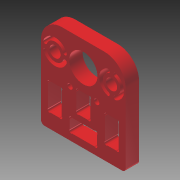
# Autodesk Inventor part: gantry2
Saved by Autodesk Inventor 2012 SP1 (Build 160190100, 190)
## iProperties
Created: 2011-10-14
Part Number: gantry2
Document SubType Name: Modeling
Designer: cramera
Density: 0.952 g/cm^3
Material: High Density Polyethylene
Mass: 45.0071 g
Surface Area: 204.192 cm^2
Volume: 47.2763 cm^3
Autodesk Inventor part; units mm, degrees
ref_plane "YZ Plane" through (0, 0, 0) normal (1, 0, 0) x (0, 1, 0)
ref_plane "XZ Plane" through (0, 0, 0) normal (0, 1, 0) x (-1, 0, 0)
ref_plane "XY Plane" through (0, 0, 0) normal (0, 0, 1) x (1, 0, 0)
derived "skeleton.ipt"
sketch "DRILL-THROUGH" plane through (0, 0, 0) normal (0, 0, 1) x (1, 0, 0)
  arc A0 (596.6867, 478.8812) -> (598.2742, 477.2937) centre (598.2742, 478.8812) ccw
  arc A1 (598.2742, 508.2817) -> (599.8617, 509.8692) centre (598.2742, 509.8692) ccw
  arc A2 (599.8617, 509.8692) -> (598.2742, 511.4567) centre (598.2742, 509.8692) ccw
  arc A3 (598.2742, 511.4567) -> (596.6867, 509.8692) centre (598.2742, 509.8692) ccw
  arc A4 (596.6867, 509.8692) -> (598.2742, 508.2817) centre (598.2742, 509.8692) ccw
  arc A5 (629.2622, 508.2817) -> (630.8497, 509.8692) centre (629.2622, 509.8692) ccw
  arc A6 (630.8497, 509.8692) -> (629.2622, 511.4567) centre (629.2622, 509.8692) ccw
  arc A7 (629.2622, 511.4567) -> (627.6747, 509.8692) centre (629.2622, 509.8692) ccw
  arc A8 (627.6747, 509.8692) -> (629.2622, 508.2817) centre (629.2622, 509.8692) ccw
  arc A9 (599.8617, 478.8812) -> (598.2742, 480.4687) centre (598.2742, 478.8812) ccw
  arc A10 (598.2742, 477.2937) -> (599.8617, 478.8812) centre (598.2742, 478.8812) ccw
  arc A11 (598.2742, 480.4687) -> (596.6867, 478.8812) centre (598.2742, 478.8812) ccw
  arc A12 (630.8497, 478.8812) -> (629.2622, 480.4687) centre (629.2622, 478.8812) ccw
  arc A13 (629.2622, 477.2937) -> (630.8497, 478.8812) centre (629.2622, 478.8812) ccw
  arc A14 (627.6747, 478.8812) -> (629.2622, 477.2937) centre (629.2622, 478.8812) ccw
  arc A15 (629.2622, 480.4687) -> (627.6747, 478.8812) centre (629.2622, 478.8812) ccw
  constraints: 32 point on circle, 16 centre point
sketch "POCKET_3-8" plane through (0, 0, 0) normal (0, 0, 1) x (1, 0, 0)
  circle A0 centre (625.7697, 474.1185) radius 6.0458
  circle A1 centre (601.7667, 474.1185) radius 6.0458
  constraints: 2 centre point
sketch "STOCK_12MM" plane through (0, 0, 0) normal (0, 0, 1) x (1, 0, 0)
  line L0 (457.2, 0) -> (914.4, 0)
  line L1 (914.4, 0) -> (914.4, 914.4)
  line L2 (914.4, 914.4) -> (457.2, 914.4)
  line L3 (457.2, 914.4) -> (457.2, 0)
  line L4 (0, 0) -> (457.2, 0)
  line L5 (457.2, 0) -> (457.2, 914.4)
  line L6 (457.2, 914.4) -> (0, 914.4)
  line L7 (0, 914.4) -> (0, 0)
  constraints: 16 end point
sketch "THROUGH-CUT" plane through (0, 0, 0) normal (0, 0, 1) x (1, 0, 0)
  arc A0 (643.0324, 504.8484) -> (640.8954, 503.359) centre (642.4829, 503.359) ccw
  line L0 (640.8954, 503.359) -> (640.8954, 503.2506)
  arc A1 (640.8954, 503.2506) -> (641.9274, 501.7635) centre (642.4829, 503.2506) ccw
  arc A2 (641.9274, 486.9869) -> (641.9274, 501.7635) centre (639.1682, 494.3752) ccw
  arc A3 (641.9274, 486.9869) -> (640.8954, 485.4998) centre (642.4829, 485.4998) ccw
  line L1 (640.8954, 485.4998) -> (640.8954, 485.3914)
  arc A4 (575.6682, 435.1284) -> (578.8432, 431.9534) centre (578.8432, 435.1284) ccw
  line L2 (578.8432, 431.9534) -> (648.6932, 431.9534)
  arc A5 (648.6932, 431.9534) -> (651.8682, 435.1284) centre (648.6932, 435.1284) ccw
  line L3 (651.8682, 435.1284) -> (651.8682, 497.5502)
  arc A6 (651.8682, 497.5502) -> (632.8182, 516.6002) centre (632.8182, 497.5502) ccw
  line L4 (632.8182, 516.6002) -> (594.7182, 516.6002)
  arc A7 (594.7182, 516.6002) -> (575.6682, 497.5502) centre (594.7182, 497.5502) ccw
  line L5 (575.6682, 497.5502) -> (575.6682, 435.1284)
  line L6 (607.6087, 473.0801) -> (607.6087, 458.2663)
  arc A8 (607.6087, 458.2663) -> (609.8537, 456.0212) centre (608.7312, 457.1437) ccw
  line L7 (609.8537, 456.0212) -> (617.6826, 456.0212)
  arc A9 (617.6826, 456.0212) -> (619.9277, 458.2663) centre (618.8051, 457.1437) ccw
  line L8 (619.9277, 458.2663) -> (619.9277, 473.0801)
  arc A10 (619.9277, 473.0801) -> (617.6826, 475.3252) centre (618.8051, 474.2027) ccw
  line L9 (617.6826, 475.3252) -> (609.8537, 475.3252)
  arc A11 (609.8537, 475.3252) -> (607.6087, 473.0801) centre (608.7312, 474.2027) ccw
  arc A12 (601.5762, 440.5485) -> (603.8212, 438.3034) centre (602.6987, 439.426) ccw
  line L10 (603.8212, 438.3034) -> (623.7151, 438.3034)
  arc A13 (623.7151, 438.3034) -> (625.9602, 440.5485) centre (624.8376, 439.426) ccw
  line L11 (625.9602, 440.5485) -> (625.9602, 448.3774)
  arc A14 (625.9602, 448.3774) -> (623.7151, 450.6224) centre (624.8376, 449.4999) ccw
  line L12 (623.7151, 450.6224) -> (603.8212, 450.6224)
  arc A15 (603.8212, 450.6224) -> (601.5762, 448.3774) centre (602.6987, 449.4999) ccw
  line L13 (601.5762, 448.3774) -> (601.5762, 440.5485)
  arc A16 (582.0182, 447.122) -> (582.0182, 444.877) centre (583.1407, 445.9995) ccw
  arc A17 (597.2436, 492.648) -> (595.7564, 491.6159) centre (597.2436, 491.0605) ccw
  line L14 (584.2632, 444.877) -> (592.0921, 444.877)
  arc A18 (592.0921, 444.877) -> (594.3372, 447.122) centre (593.2146, 445.9995) ccw
  line L15 (594.3372, 447.122) -> (594.3372, 467.0159)
  arc A19 (594.3372, 467.0159) -> (592.0921, 469.261) centre (593.2146, 468.1384) ccw
  line L16 (592.0921, 469.261) -> (584.2632, 469.261)
  arc A20 (584.2632, 469.261) -> (582.0182, 469.261) centre (583.1407, 468.1384) ccw
  arc A21 (582.0182, 469.261) -> (582.0182, 467.0159) centre (583.1407, 468.1384) ccw
  line L17 (582.0182, 467.0159) -> (582.0182, 447.122)
  arc A22 (633.1992, 447.122) -> (635.4442, 444.877) centre (634.3217, 445.9995) ccw
  line L18 (635.4442, 444.877) -> (643.2731, 444.877)
  arc A23 (643.2731, 444.877) -> (645.5182, 447.122) centre (644.3956, 445.9995) ccw
  line L19 (645.5182, 447.122) -> (645.5182, 467.0159)
  arc A24 (645.5182, 467.0159) -> (643.2731, 469.261) centre (644.3956, 468.1384) ccw
  line L20 (643.2731, 469.261) -> (635.4442, 469.261)
  arc A25 (635.4442, 469.261) -> (633.1992, 467.0159) centre (634.3217, 468.1384) ccw
  line L21 (633.1992, 467.0159) -> (633.1992, 447.122)
  arc A26 (601.0682, 494.3752) -> (613.7682, 481.6752) centre (613.7682, 494.3752) ccw
  arc A27 (613.7682, 481.6752) -> (626.4682, 494.3752) centre (613.7682, 494.3752) ccw
  arc A28 (626.4682, 494.3752) -> (613.7682, 507.0752) centre (613.7682, 494.3752) ccw
  arc A29 (613.7682, 507.0752) -> (601.0682, 494.3752) centre (613.7682, 494.3752) ccw
  arc A30 (601.7667, 476.5315) -> (599.3537, 474.1185) centre (601.7667, 474.1185) ccw
  arc A31 (599.3537, 474.1185) -> (601.7667, 471.7055) centre (601.7667, 474.1185) ccw
  arc A32 (601.7667, 471.7055) -> (604.1797, 474.1185) centre (601.7667, 474.1185) ccw
  arc A33 (604.1797, 474.1185) -> (601.7667, 476.5315) centre (601.7667, 474.1185) ccw
  arc A34 (597.352, 496.1024) -> (598.8413, 498.2394) centre (597.352, 497.6899) ccw
  arc A35 (598.8413, 498.2394) -> (577.895, 498.2394) centre (588.3682, 494.3752) ccw
  arc A36 (577.895, 498.2394) -> (579.3844, 496.1024) centre (579.3844, 497.6899) ccw
  line L22 (579.3844, 496.1024) -> (579.4927, 496.1024)
  arc A37 (625.7697, 476.5315) -> (623.3567, 474.1185) centre (625.7697, 474.1185) ccw
  arc A38 (623.3567, 474.1185) -> (625.7697, 471.7055) centre (625.7697, 474.1185) ccw
  arc A39 (625.7697, 471.7055) -> (628.1827, 474.1185) centre (625.7697, 474.1185) ccw
  arc A40 (628.1827, 474.1185) -> (625.7697, 476.5315) centre (625.7697, 474.1185) ccw
  circle A41 centre (639.1682, 494.3752) radius 5
  arc A42 (579.4927, 496.1024) -> (580.9799, 497.1345) centre (579.4927, 497.6899) ccw
  arc A43 (595.7564, 497.1345) -> (580.9799, 497.1345) centre (588.3682, 494.3752) ccw
  arc A44 (595.7564, 497.1345) -> (597.2436, 496.1024) centre (597.2436, 497.6899) ccw
  line L23 (597.2436, 496.1024) -> (597.352, 496.1024)
  circle A45 centre (588.3682, 494.3752) radius 5
  arc A46 (598.8413, 490.511) -> (597.352, 492.648) centre (597.352, 491.0605) ccw
  arc A47 (577.895, 490.511) -> (598.8413, 490.511) centre (588.3682, 494.3752) ccw
  arc A48 (579.3844, 492.648) -> (577.895, 490.511) centre (579.3844, 491.0605) ccw
  arc A49 (582.0182, 444.877) -> (584.2632, 444.877) centre (583.1407, 445.9995) ccw
  line L24 (579.3844, 492.648) -> (579.4927, 492.648)
  arc A50 (580.9799, 491.6159) -> (579.4927, 492.648) centre (579.4927, 491.0605) ccw
  arc A51 (580.9799, 491.6159) -> (595.7564, 491.6159) centre (588.3682, 494.3752) ccw
  line L25 (597.2436, 492.648) -> (597.352, 492.648)
  arc A52 (637.441, 503.359) -> (635.3039, 504.8484) centre (635.8535, 503.359) ccw
  line L26 (637.441, 503.359) -> (637.441, 503.2506)
  arc A53 (636.4089, 501.7635) -> (637.441, 503.2506) centre (635.8535, 503.2506) ccw
  arc A54 (636.4089, 501.7635) -> (636.4089, 486.9869) centre (639.1682, 494.3752) ccw
  arc A55 (637.441, 485.4998) -> (636.4089, 486.9869) centre (635.8535, 485.4998) ccw
  line L27 (637.441, 485.4998) -> (637.441, 485.3914)
  arc A56 (635.3039, 483.902) -> (637.441, 485.3914) centre (635.8535, 485.3914) ccw
  arc A57 (635.3039, 504.8484) -> (635.3039, 483.902) centre (639.1682, 494.3752) ccw
  arc A58 (640.8954, 485.3914) -> (643.0324, 483.902) centre (642.4829, 485.3914) ccw
  arc A59 (643.0324, 483.902) -> (643.0324, 504.8484) centre (639.1682, 494.3752) ccw
  dimension "d5" = 10
  dimension "d6" = 10
  constraints: 116 point on circle, 60 centre point, 56 end point
  measures "d5" diameter of A45
  measures "d6" diameter of A41
extrude "Extrusion1" add sketch "THROUGH-CUT" along normal blind 12
extrude "Extrusion2" cut sketch "POCKET_3-8" along normal blind 9.525
equation "\"d6\" = d5"
equation "\"d1\" = StockThickness"
equation "\"StockThickness\" = 12"
body "Solid1"
